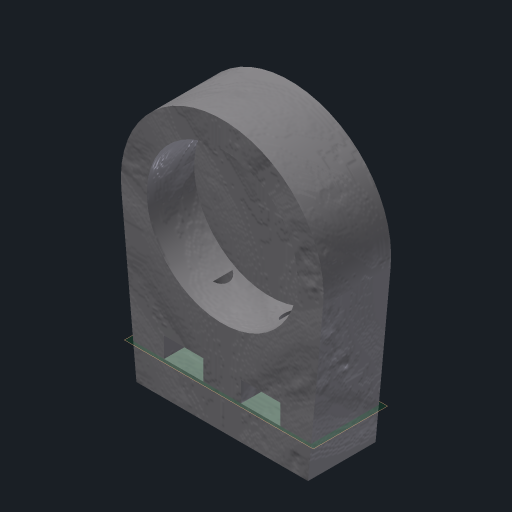
# Autodesk Inventor part: OTRO_EXTREMO
Saved by Autodesk Inventor 2024.3 (Build 283343000, 343)
## iProperties
Created: 2024-08-24
Part Number: OTRO_EXTREMO
Material: Steel, Mild, Welded
Document SubType Name: Modeling
Designer: Niler
Density: 7.85 g/cm^3
Appearance: Weld - Steel Mild
Author: Niler
Autodesk Inventor part; units mm, degrees
ref_plane "YZ Plane" through (0, 0, 0) normal (1, 0, 0) x (0, 1, 0)
ref_plane "XZ Plane" through (0, 0, 0) normal (0, 1, 0) x (-1, 0, 0)
ref_plane "XY Plane" through (0, 0, 0) normal (0, 0, 1) x (1, 0, 0)
sketch "Sketch1" plane through (0, 0, 0) normal (0, 0, 1) x (1, 0, 0)
  circle A0 centre (0, 25) radius 4.1
  circle A1 centre (0, 25) radius 15
  line L0 (-14.9332, 23.5861) -> (-12.7, 0)
  line L1 (-12.7, 0) -> (0, 0)
  line L2 (0, 0) -> (0, 25)
  line L3 (14.9332, 23.5861) -> (12.7, 0)
  line L4 (12.7, 0) -> (0, 0)
  circle A2 centre (0, 25) radius 11.15
  point P0 (14.9332, 23.5861)
  dimension "d1" = 30
  dimension "d0" = 8.2
  dimension "d2" = 25.4
  dimension "d5" = 25
  dimension "d16" = 22.3
  constraints: 10 end point, 2 centre point, 2 coincident, 2 symmetric about line, 1 horizontal, 1 perpendicular, 4 other
  measures "d0" diameter of A0
  measures "d2" distance of L3.end L0.end
  measures "d5" distance from line of L1 A0.centre
  measures "d16" diameter of A2
extrude "Extrusion1" add sketch "Sketch1" along normal blind 10 contours A2 | A1 | A1 L3 L4 L2 | L2 L1 L0 A1
sketch "Sketch2" plane through (-12.7, 0, 0) normal (0, -1, 0) x (1, 0, 0)
  line L0 (0, 0) -> (25.4, 0) projected
  line L1 (25.4, 0) -> (25.4, 10) projected
  line L2 (0, 10) -> (25.4, 10) projected
  line L3 (0, 0) -> (0, 10) projected
  circle A0 centre (7, 5) radius 1.65
  point P0 (12.7, 0)
  point P1 (0, 5)
  dimension "d6" = 3.3
  dimension "d7" = 7
  constraints: 1 centre point, 1 horizontal alignment, 1 midpoint
  measures "d6" diameter of A0
  measures "d7" distance from line of L3 A0.centre
extrude "Extrusion2" cut sketch "Sketch2" against normal blind 15 contours A0
ref_plane "Work Plane1" through (-12.7, 5, 0) normal (0, -1, 0) x (1, 0, 0)
sketch "Sketch3" plane through (-12.7, 5, 0) normal (0, -1, 0) x (1, 0, 0)
  circle A0 centre (7, 5) radius 1.65 projected
  line L0 (9.9, 6.6743) -> (9.9, 3.3257)
  line L1 (9.9, 3.3257) -> (7, 1.6514)
  line L2 (7, 1.6514) -> (4.1, 3.3257)
  line L3 (4.1, 3.3257) -> (4.1, 6.6743)
  line L4 (4.1, 6.6743) -> (7, 8.3486)
  line L5 (7, 8.3486) -> (9.9, 6.6743)
  line L6 (4.1, 6.6743) -> (9.9, 6.6743)
  line L7 (9.9, 6.6743) -> (9.9, 13.9222)
  line L8 (9.9, 13.9222) -> (4.1, 13.9222)
  line L9 (4.1, 13.9222) -> (4.1, 6.6743)
  point P0 (12.7, 0)
  dimension "d11" = 5.8
  constraints: 20 end point, 2 parallel, 1 coincident, 1 horizontal, 1 perpendicular, 1 vertical alignment, 13 other
  measures "d11" distance between parallel lines of L0 L3
extrude "Extrusion3" cut sketch "Sketch3" against normal blind 3
mirror "Mirror1" about plane through (0, 0, 0) normal (1, 0, 0) of "Extrusion3", "Extrusion2"
sketch "Sketch4" plane through (0, 0, 0) normal (0, 0, -1) x (-1, 0, 0)
  line L0 (12.7, 0) -> (-12.7, 0) projected
  line L1 (14.9332, 23.5861) -> (12.7, 0) projected
  arc A0 (14.9332, 23.5861) -> (-14.9332, 23.5861) centre (0, 25) ccw projected
  line L2 (-12.7, 0) -> (-14.9332, 23.5861) projected
  circle A1 centre (0, 25) radius 4.1 projected
  point P0 (0, 0)
extrude "Extrusion4" add sketch "Sketch4" against normal blind 3 contours A1
sketch "Sketch5" plane through (0, 0, 10) normal (0, 0, 1) x (1, 0, 0)
  line L0 (8.6, 8) -> (8.6, 5) projected
  line L1 (8.6, 5) -> (2.8, 5) projected
  line L2 (2.8, 5) -> (2.8, 8) projected
  line L3 (2.8, 8) -> (8.6, 8) projected
  line L4 (-8.6, 5) -> (-8.6, 8) projected
  line L5 (-8.6, 8) -> (-2.8, 8) projected
  line L6 (-2.8, 8) -> (-2.8, 5) projected
  line L7 (-2.8, 5) -> (-8.6, 5) projected
  line L8 (-12.7, 0) -> (12.7, 0) projected
  line L9 (12.7, 0) -> (14.9332, 23.5861) projected
  arc A0 (14.9332, 23.5861) -> (-14.9332, 23.5861) centre (0, 25) ccw projected
  line L10 (-14.9332, 23.5861) -> (-12.7, 0) projected
  circle A1 centre (0, 25) radius 4.1 projected
  circle A2 centre (0, 25) radius 4.1 projected
  circle A3 centre (0, 25) radius 11.15
  point P0 (0, 0)
  dimension "d17" = 22.3
  constraints: 1 centre point, 1 coincident
  measures "d17" diameter of A3
extrude "Extrusion5" cut sketch "Sketch5" against normal blind 7 contours A3
body "Solid1"
